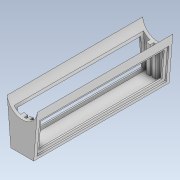
# Autodesk Inventor part: Tractive Light Mount
Saved by Autodesk Inventor 2021 (Build 250183000, 183)
## iProperties
Created: 2020-09-26
Part Number: Tractive Light Mount
Material: Generic
Document SubType Name: Modeling
Designer: capta
Density: 1 g/cm^3
Appearance: Default
Author: capta
Autodesk Inventor part; units mm, degrees
ref_plane "YZ Plane" through (0, 0, 0) normal (1, 0, 0) x (0, 1, 0)
ref_plane "XZ Plane" through (0, 0, 0) normal (0, 1, 0) x (-1, 0, 0)
ref_plane "XY Plane" through (0, 0, 0) normal (0, 0, 1) x (1, 0, 0)
sketch "Sketch1" plane through (0, 0, 0) normal (0, 0, 1) x (1, 0, 0)
  arc A0 (-12.6587, -1.0228) -> (12.6587, -1.0228) centre (0, 0) ccw
  line L0 (0, 0) -> (0, -38.1)
  line L1 (0, -38.1) -> (-9.663, -38.1)
  line L2 (-9.663, -38.1) -> (-12.6587, -1.0228)
  line L3 (0, -38.1) -> (9.663, -38.1)
  line L4 (9.663, -38.1) -> (12.6587, -1.0228)
  dimension "d0" = 25.4
  dimension "d1" = 38.1
  dimension "d2" = 9.663
  dimension "d3" = 9.663
  constraints: 10 end point, 2 point on circle, 2 tangent, 1 centre point, 1 coincident, 1 horizontal, 1 point on line, 1 vertical
  measures "d0" diameter of A0
  measures "d1" distance of L0.start L0.end
  measures "d2" distance of L0.end L1.end
  measures "d3" distance of L0.end L3.end
extrude "Extrusion1" add sketch "Sketch1" along normal blind 114.3
shell "Shell1" thickness 2.54 removed faces 1 at (-12.5308, -2.0661, 76.2)
sketch "Sketch2" plane through (-9.5133, -8.4135, 111.76) normal (0.9967519, 0.0805339, 0) x (0, 0, -1)
  line L0 (109.22, 0) -> (109.22, -27.235) projected
  line L1 (0, 0) -> (109.22, 0) projected
  line L2 (0, 0) -> (0, -27.235) projected
  line L3 (109.22, -27.235) -> (0, -27.235) projected
  line L4 (106.68, -2.54) -> (106.68, -24.695)
  line L5 (106.68, -24.695) -> (2.54, -24.695)
  line L6 (2.54, -24.695) -> (2.54, -2.54)
  line L7 (2.54, -2.54) -> (106.68, -2.54)
  point P0 (111.76, 7.62)
  dimension "d9" = 2.54
  constraints: 8 end point, 3 other
  measures "d9" distance between parallel lines of L1 L7
sketch "Sketch3" plane through (-9.663, -38.1, 0) normal (-0.9967519, -0.0805339, 0) x (0, 0, 1)
  line L0 (2.54, 29.578) -> (2.54, 2.3431) projected
  line L1 (111.76, 29.578) -> (2.54, 29.578) projected
  line L2 (111.76, 29.578) -> (111.76, 2.3431) projected
  line L3 (2.54, 2.3431) -> (111.76, 2.3431) projected
  point P0 (0, 37.198)
extrude "Extrusion2" cut sketch "Sketch3" against normal blind 1.27
extrude "Extrusion3" cut sketch "Sketch2" against normal blind 1.27 contours L4 L5 L6 L7
mirror "Mirror1" about plane through (0, 0, 0) normal (1, 0, 0) of "Extrusion3", "Extrusion2"
sketch "Sketch4" plane through (-7.32, -35.56, 2.54) normal (0, 1, 0) x (1, 0, 0)
  line L0 (16.8333, -109.22) -> (-2.1933, -109.22) projected
  line L1 (7.32, -109.22) -> (6.431, -109.22)
  line L2 (6.431, -109.22) -> (6.431, -106.172)
  line L3 (6.431, -106.172) -> (3.383, -106.172)
  line L4 (3.383, -106.172) -> (3.383, -109.22)
  line L5 (-2.1933, -109.22) -> (16.8333, -109.22)
  line L6 (7.32, -109.22) -> (8.209, -109.22)
  line L7 (8.209, -109.22) -> (8.209, -106.172)
  line L8 (8.209, -106.172) -> (11.257, -106.172)
  line L9 (11.257, -106.172) -> (11.257, -109.22)
  point P0 (7.32, 2.54)
  dimension "d12" = 0.889
  dimension "d13" = 3.048
  dimension "d14" = 3.048
  constraints: 18 end point, 4 point on line, 1 horizontal, 1 midpoint, 1 perpendicular, 1 vertical
  measures "d12" distance of L1.start L1.end
  measures "d13" distance of L1.end L2.end
  measures "d14" distance of L2.end L3.end
extrude "Extrusion4" add sketch "Sketch4" along normal blind 26.67
ref_plane "Work Plane1" through (0, 0, 57.15) normal (0, 0, -1) x (-1, 0, 0)
mirror "Mirror2" about plane through (0, 0, 57.15) normal (0, 0, -1) of "Extrusion4"
sketch "Sketch6" plane through (0, 0, 0) normal (0, 0, -1) x (-1, 0, 0)
  arc A0 (-12.6587, -1.0228) -> (12.6587, -1.0228) centre (0, 0) ccw projected
  line L0 (-12.6587, -1.0228) -> (12.6587, -1.0228)
  constraints: 2 end point, 1 horizontal
extrude "Extrusion6" cut sketch "Sketch6" against normal blind 304.8
body "Solid1"
